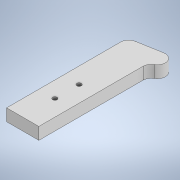
# Autodesk Inventor part: remoteswitchtouch
Saved by Autodesk Inventor 2021 (Build 250183000, 183)
## iProperties
Created: 2021-10-25
Part Number: remoteswitchtouch
Material: Generic
Document SubType Name: Modeling
Designer: eddys
Density: 1 g/cm^3
Appearance: Default
Author: eddys
Autodesk Inventor part; units mm, degrees
ref_plane "YZ Plane" through (0, 0, 0) normal (1, 0, 0) x (0, 1, 0)
ref_plane "XZ Plane" through (0, 0, 0) normal (0, 1, 0) x (-1, 0, 0)
ref_plane "XY Plane" through (0, 0, 0) normal (0, 0, 1) x (1, 0, 0)
sketch "Sketch1" plane through (0, 0, 0) normal (0, 1, 0) x (-1, 0, 0)
  line L0 (4.0096, 14.964) -> (-3.9904, 14.964)
  line L1 (-3.9904, 14.964) -> (-3.9904, -12.0894)
  line L2 (4.0096, -15.036) -> (4.0096, 14.964)
  line L3 (4.0096, 14.964) -> (-4.018, -14.9952) construction
  line L4 (-3.9904, 14.964) -> (4.0096, -15.036) construction
  line L5 (4.0096, -15.036) -> (-6.0407, -16.8081)
  line L6 (-3.9904, -12.0894) -> (-6.4901, -13.5325)
  line L7 (-6.4901, -13.5325) -> (-6.0407, -16.8081)
  point P0 (0, 0)
  dimension "d5" = 30
  dimension "d6" = 8
  dimension "d7" = 7.812
  dimension "d8" = 120
  dimension "d9" = 100
  dimension "d10" = 3.2756
  dimension "d11" = 27.0534
  dimension "d12" = 45
  constraints: 16 end point, 2 point on line, 1 horizontal, 1 parallel, 1 perpendicular
  measures "d5" distance of L2.start L0.start
  measures "d6" distance of L0.start L0.end
  measures "d7" angle of L7 L2
  measures "d8" angle of L1 L6
  measures "d9" angle of L5 L2
  measures "d10" vertical distance of L6.end L5.end
  measures "d11" distance of L0.end L1.end
  measures "d12" angle of L3 L6
extrude "Extrusion1" add sketch "Sketch1" along normal blind 3
fillet "Fillet1" radius 2 4 edges at (-4.0096, 1.5, -15.036) (6.0407, 1.5, -16.8081) (6.4901, 1.5, -13.5325) (3.9904, 1.5, -12.0894)
sketch "Sketch2" plane through (0, 3, 0) normal (0, 1, 0) x (1, 0, 0)
  circle A0 centre (-0.0096, -6.964) radius 0.55
  line L0 (-4.0096, -14.964) -> (3.9904, -14.964) projected
  line L1 (-4.0096, 13.3578) -> (-4.0096, -14.964) projected
  circle A1 centre (-0.0096, -0.964) radius 0.55
  point P0 (0, 0)
  dimension "d16" = 8
  dimension "d17" = 1.1
  dimension "d18" = 4
  dimension "d19" = 14
  dimension "d20" = 4
  dimension "d21" = 1.1
  constraints: 2 centre point
  measures "d16" distance from line of L0 A0.centre
  measures "d17" diameter of A0
  measures "d18" distance from line of L1 A0.centre
  measures "d19" distance from line of L0 A1.centre
  measures "d20" distance from line of L1 A1.centre
  measures "d21" diameter of A1
extrude "Extrusion2" cut sketch "Sketch2" against normal blind 3
body "Solid1"
